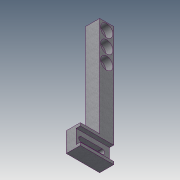
# Autodesk Inventor part: J005772
Saved by Autodesk Inventor 2015 SP1 (Build 190203100, 203)
## iProperties
Created: 2009-02-23
Part Number: J005772
Document SubType Name: Modeling
Designer: xun
Density: 7.8 g/cm^3
Material: STAINLESS STEEL, 17-4, H900
Appearance: Metal-Steel (Stainless, Brushed)
Description: MOUSE LEFT HEADBAR BASE
Project: COMMON
Vendor: HHMI: JRC - ID&F
ALTERED ITEM PART NUMBER: N/A
ALTERED ITEM VENDOR: N/A
SPECIAL FINISH: NONE
SURFACE ROUGHNESS: 63 Ra
LAB/DEPT: COMMON
REQUESTING SCIENTIST: COMMON
DESIGN DEPARTMENT: HHMI: JRC - ID&F
ALTERED ITEM DESCRIPTION: N/A
Author: xun
Revision Number: -
Autodesk Inventor part; units mm, degrees
ref_plane "YZ Plane" through (0, 0, 0) normal (1, 0, 0) x (0, 1, 0)
ref_plane "XZ Plane" through (0, 0, 0) normal (0, 1, 0) x (-1, 0, 0)
ref_plane "XY Plane" through (0, 0, 0) normal (0, 0, 1) x (1, 0, 0)
sketch "Sketch1" plane through (0, 0, 0) normal (0, 0, 1) x (1, 0, 0)
  line L0 (3.0839, 107.4917) -> (15.7839, 107.4917)
  line L1 (15.7839, 107.4917) -> (15.7839, -0.4583)
  line L2 (15.7839, -0.4583) -> (3.0839, -0.4583)
  line L3 (3.0839, -0.4583) -> (3.0839, 107.4917)
  line L4 (33.221, 2.0817) -> (3.0839, 2.0817)
  line L5 (33.221, 14.8071) -> (3.0839, 14.8071)
  line L6 (15.7839, -0.4583) -> (33.221, -0.4583)
  line L7 (33.221, -0.4583) -> (33.221, 17.3471)
  line L8 (33.221, 17.3471) -> (15.7839, 17.3471)
  circle A0 centre (28.776, 8.4444) radius 2.159
  circle A1 centre (9.726, 8.4444) radius 2.159
  line L9 (9.726, 6.2854) -> (28.776, 6.2854)
  line L10 (9.726, 10.6034) -> (28.776, 10.6034)
  point P0 (9.4212, 101.1417)
  point P1 (9.4212, 88.4417)
  point P2 (9.4212, 75.7417)
  point P3 (15.7839, 2.0817)
  point P4 (15.7839, 14.8071)
  dimension "d0" = 12.7
  dimension "d1" = 107.95
  dimension "d2" = 6.35
  dimension "d3" = 12.7
  dimension "d4" = 6.3626
  dimension "d5" = 6.3626
  dimension "d6" = 6.3626
  dimension "d7" = 12.7
  dimension "d17" = 2.54
  dimension "d18" = 12.7254
  dimension "d21" = 17.4371
  dimension "d22" = 2.54
  dimension "d23" = 4.318
  dimension "d24" = 6.3627
  dimension "d25" = 4.445
  dimension "d26" = 4.318
  dimension "d27" = 6.3627
  dimension "d28" = 19.05
  constraints: 22 end point, 9 point on line, 5 perpendicular, 4 parallel, 4 point on circle, 3 tangent, 2 centre point, 1 horizontal
  measures "d0" distance of L0.start L0.end
  measures "d1" distance of L0.end L1.end
  measures "d2" distance from line of L0 point (9.421, 101.142)
  measures "d3" distance of point (9.421, 88.442) point (9.421, 101.142)
  measures "d4" distance from line of L1 point (9.421, 101.142)
  measures "d5" distance from line of L1 point (9.421, 88.442)
  measures "d6" distance from line of L1 point (9.421, 75.742)
  measures "d7" distance of point (9.421, 75.742) point (9.421, 88.442)
  measures "d17" distance between parallel lines of L4 L2
  measures "d18" distance between parallel lines of L4 L5
  measures "d21" distance of L1.end L6.end
  measures "d22" distance between parallel lines of L5 L8
  measures "d23" diameter of A0
  measures "d24" distance from line of L4 A0.centre
  measures "d25" distance from line of L7 A0.centre
  measures "d26" diameter of A1
  measures "d27" distance from line of L4 A1.centre
  measures "d28" distance of A0.centre A1.centre
extrude "Extrusion1" add sketch "Sketch1" along normal blind 12.7
hole "Hole1" at (9.4212, 101.1417, 0) at (9.4212, 88.4417, 0) at (9.4212, 75.7417, 0) direction (0, 0, 1) diameter 6.5278 end through all counterbore diameter 11.1252 counterbore depth 6.35 clearance for "Socket Head Cap Screw" size "1/4" standard "Ansi Unified Screw Threads"
extrude "Extrusion2" cut sketch "Sketch1" along normal blind 3.81 contours L5 L1 L10 A1 L9 L4 L3 | L5 L7 L4 L1 L9 A0 L10 | L10 A0 L9 L1 | L1 L9 A1 L10 | A1 | A0
extrude "Extrusion3" cut sketch "Sketch1" along normal through all contours L10 A0 L9 L1 | L1 L9 A1 L10 | A1 | A0
equation "\"d29\" = d27"
body "Solid1"
